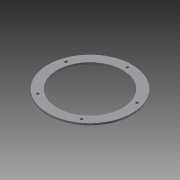
# Autodesk Inventor part: HeatingElementHolder01
Saved by Autodesk Inventor 2015 (Build 190159000, 159)
## iProperties
Created: 2016-08-08
Part Number: HeatingElementHolder01
Material: Generic
Document SubType Name: Modeling
Designer: spichelh
Density: 1 g/cm^3
Appearance: Default
Author: spichelh
Autodesk Inventor part; units mm, degrees
ref_plane "YZ Plane" through (0, 0, 0) normal (1, 0, 0) x (0, 1, 0)
ref_plane "XZ Plane" through (0, 0, 0) normal (0, 1, 0) x (-1, 0, 0)
ref_plane "XY Plane" through (0, 0, 0) normal (0, 0, 1) x (1, 0, 0)
sketch "Sketch1" plane through (0, 0, 0) normal (0, 1, 0) x (-1, 0, 0)
  circle A0 centre (0, 0) radius 45
  circle A1 centre (0, 0) radius 35
  dimension "d0" = 10
  dimension "d1" = 70
  constraints: 2 centre point, 2 coincident
  measures "d0" radial gap between concentric circles of A0 A1
  measures "d1" diameter of A1
extrude "Extrusion1" add sketch "Sketch1" along normal blind 2
sketch "Sketch2" plane through (0, 2, 0) normal (0, 1, 0) x (1, 0, 0)
  circle A0 centre (0, 40) radius 1.5
  line L0 (0, 0) -> (0, 64.6181) construction
  circle A1 centre (-38.0423, 12.3607) radius 1.5
  line L1 (0, 0) -> (-61.4554, 19.9681) construction
  circle A2 centre (-23.5114, -32.3607) radius 1.5
  line L2 (0, 0) -> (-37.9816, -52.2771) construction
  circle A3 centre (23.5114, -32.3607) radius 1.5
  line L3 (0, 0) -> (37.9816, -52.2771) construction
  circle A4 centre (38.0423, 12.3607) radius 1.5
  line L4 (0, 0) -> (61.4554, 19.9681) construction
  dimension "d4" = 3
  dimension "d5" = 40
  dimension "d8" = 360
  constraints: 10 end point, 5 centre point, 5 point on line, 1 coincident, 1 vertical, 26 other
  measures "d4" diameter of A0
  measures "d5" distance of A0.centre L0.start
extrude "Extrusion2" cut sketch "Sketch2" against normal blind 3
body "Solid1"
